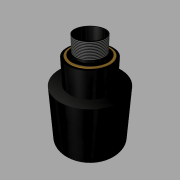
# Autodesk Inventor part: M12 2.8-12mm F1.4 Lens
Saved by Autodesk Inventor 2019 (Build 230136000, 136)
## iProperties
Created: 2019-05-09
Part Number: M12 2.8-12mm F1.4 Lens
Material: Generic
Document SubType Name: Modeling
Designer: Ben
Density: 1 g/cm^3
Appearance: Default
Author: Ben
Autodesk Inventor part; units mm, degrees
sketch "Sketch1" plane through (0, 0, 0) normal (0, 1, 0) x (-1, 0, 0)
  circle A0 centre (0, 0) radius 5.925
  circle A1 centre (0, 0) radius 5.325
  dimension "d0" = 11.85
  dimension "d1" = 0.6
  constraints: 2 centre point, 1 coincident
  measures "d0" diameter of A0
  measures "d1" radial gap between concentric circles of A0 A1
extrude "Extrusion1" add sketch "Sketch1" against normal blind 7
thread "Thread1" size "M12x0.5" class "6g" standard "ANSI Metric M Profile" length 6 offset 1
sketch "Sketch2" plane through (0, -7, 0) normal (0, -1, 0) x (1, 0, 0)
  circle A0 centre (0, 0) radius 7.5
  circle A1 centre (0, 0) radius 5.325 projected
  dimension "d6" = 15
  constraints: 1 centre point, 1 coincident
  measures "d6" diameter of A0
extrude "Extrusion2" add sketch "Sketch2" along normal blind 0.25
sketch "Sketch3" plane through (0, -7.25, 0) normal (0, -1, 0) x (1, 0, 0)
  circle A0 centre (0, 0) radius 8.375
  circle A1 centre (0, 0) radius 6.5
  dimension "d9" = 16.75
  dimension "d10" = 13
  constraints: 2 centre point, 2 coincident
  measures "d9" diameter of A0
  measures "d10" diameter of A1
extrude "Extrusion3" add sketch "Sketch3" along normal blind 0.25 separate body
sketch "Sketch4" plane through (0, -7.25, 0) normal (0, -1, 0) x (1, 0, 0)
  circle A0 centre (0, 0) radius 5.325 projected
  circle A1 centre (0, 0) radius 6.5 projected
extrude "Extrusion4" add sketch "Sketch4" along normal blind 0.25 bodies 1
sketch "Sketch5" plane through (0, -7.5, 0) normal (0, -1, 0) x (1, 0, 0)
  circle A0 centre (0, 0) radius 5.325 projected
  circle A1 centre (0, 0) radius 9.5
  dimension "d15" = 19
  constraints: 1 centre point, 1 coincident
  measures "d15" diameter of A1
extrude "Extrusion5" add sketch "Sketch5" along normal blind 10.5 bodies 1
sketch "Sketch6" plane through (0, -18, 0) normal (0, -1, 0) x (1, 0, 0)
  circle A0 centre (0, 0) radius 14.25
  circle A1 centre (0, 0) radius 9.5 construction
  circle A2 centre (0, 0) radius 8.5
  dimension "d18" = 28.5
  dimension "d19" = 1
  constraints: 2 centre point, 1 coincident
  measures "d18" diameter of A0
  measures "d19" radial gap between concentric circles of A1 A2
extrude "Extrusion6" add sketch "Sketch6" along normal blind 4 bodies 1
sketch "Sketch7" plane through (0, -22, 0) normal (0, -1, 0) x (1, 0, 0)
  circle A0 centre (0, 0) radius 14.25 projected
  circle A1 centre (0, 0) radius 12.75
  dimension "d22" = 1.5
  constraints: 1 centre point
  measures "d22" radial gap between concentric circles of A0 A1
extrude "Extrusion7" add sketch "Sketch7" along normal blind 20 bodies 1
ref_plane "Large Optic" through (0, -37, 0) normal (0, -1, 0) x (1, 0, 0)
sketch "Sketch8" plane through (0, -37, 0) normal (0, -1, 0) x (1, 0, 0)
  circle A0 centre (0, 0) radius 12.75 construction
  circle A1 centre (0, 0) radius 12.6
  circle A2 centre (0, 0) radius 11.1
  dimension "d26" = 0.15
  dimension "d27" = 1.5
  constraints: 2 centre point
  measures "d26" radial gap between concentric circles of A0 A1
  measures "d27" radial gap between concentric circles of A1 A2
extrude "Extrusion8" add sketch "Sketch8" against normal blind 4 separate body
ref_plane "Large Optic Lens" through (0, -35, 0) normal (0, -1, 0) x (1, 0, 0)
sketch "Sketch9" plane through (0, -35, 0) normal (0, -1, 0) x (1, 0, 0)
  circle A0 centre (0, 0) radius 11.1 projected
sketch "Sketch10" plane through (0, 0, 0) normal (1, 0, 0) x (0, 1, 0)
  line L0 (-35, 11.1) -> (-35, -11.1) construction
  line L1 (-35, 0) -> (-36.333, 0)
  arc A0 (-35, 11.1) -> (-36.333, 0) centre (10.5488, 0) ccw
  line L2 (-35, 11.1) -> (-35, 0)
  point P0 (0, 0)
  dimension "d30" = 1.333
  constraints: 4 end point, 2 point on circle, 1 centre point, 1 collinear, 1 horizontal, 1 midpoint, 1 point on line
  measures "d30" distance of L1.start L1.end
revolve "Revolution1" add sketch "Sketch10" angle 360 about axis through (0, -35, 0) along (0, -1, 0) separate body
ref_plane "Small Optic Lens" through (0, -17.5, 0) normal (0, -1, 0) x (1, 0, 0)
sketch "Sketch12" plane through (0, 0, 0) normal (1, 0, 0) x (0, 1, 0)
  line L0 (-17.5, -19.95) -> (-17.5, 19.95) construction
  line L1 (-17.5, 0) -> (-16.5, 0)
  arc A0 (-16.5, 0) -> (-17.5, 5.325) centre (-31.1778, 0) ccw
  line L2 (0, 5.325) -> (-18, 5.325) construction
  line L3 (-17.5, 0) -> (-17.5, 5.325)
  point P0 (0, 0)
  dimension "d33" = 1
  constraints: 4 end point, 3 point on line, 2 perpendicular, 2 point on circle, 1 centre point, 1 midpoint
  measures "d33" distance of L1.start L1.end
revolve "Revolution2" add sketch "Sketch12" angle 360 about axis through (0, -17.5, 0) along (0, 1, 0) bodies 4
body "Solid1"
body "Solid2"
body "Solid3"
body "Solid4"
